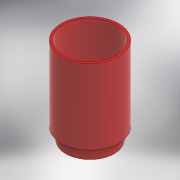
# Autodesk Inventor part: flour_duct
Saved by Autodesk Inventor 2020 (Build 240168000, 168)
## iProperties
Created: 2020-06-18
Part Number: flour_duct
Material: Generic
Document SubType Name: Modeling
Designer: pc-konvi
Density: 1 g/cm^3
Appearance: Red
Author: pc-konvi
Autodesk Inventor part; units mm, degrees
ref_plane "YZ Plane" through (0, 0, 0) normal (1, 0, 0) x (0, 1, 0)
ref_plane "XZ Plane" through (0, 0, 0) normal (0, 1, 0) x (-1, 0, 0)
ref_plane "XY Plane" through (0, 0, 0) normal (0, 0, 1) x (1, 0, 0)
sketch "Sketch1" plane through (0, 0, 0) normal (0, 0, 1) x (1, 0, 0)
  line L0 (0, 0) -> (25, 0) construction
  line L1 (25, 0) -> (25, 65) construction
  line L2 (25, 65) -> (0, 65) construction
  line L3 (0, 65) -> (0, 0) construction
  line L4 (25, 65) -> (23, 65)
  line L5 (23, 65) -> (23, 0)
  line L6 (23, 0) -> (25, 0)
  line L7 (25, 0) -> (25, 65)
  line L8 (0, 0) -> (21, 0) construction
  line L9 (21, 0) -> (21, -10) construction
  line L10 (21, -10) -> (0, -10) construction
  line L11 (0, -10) -> (0, 0) construction
  line L12 (21, 0) -> (19, 0)
  line L13 (19, 0) -> (19, -10)
  line L14 (19, -10) -> (21, -10)
  line L15 (21, -10) -> (21, 0)
  line L16 (19, 0) -> (25, 0)
  line L17 (25, 0) -> (25, 2)
  line L18 (25, 2) -> (19, 2)
  line L19 (19, 2) -> (19, 0)
  point P0 (23, 2)
  dimension "d0" = 25
  dimension "d1" = 65
  dimension "d2" = 2
  dimension "d3" = 21
  dimension "d4" = 10
  dimension "d5" = 2
  dimension "d6" = 2
  constraints: 40 end point, 10 parallel, 5 horizontal, 5 perpendicular, 3 point on line
  measures "d0" distance of L2.end L1.end
  measures "d1" distance of L1.end L0.end
  measures "d2" distance of L6.end L5.end
  measures "d3" distance of L9.end L10.end
  measures "d4" distance of L8.end L9.end
  measures "d5" distance of L14.end L13.end
  measures "d6" distance of L17.end L16.end
revolve "Revolution1" add sketch "Sketch1" angle 360 about axis through (0, 65, 0) along (0, -1, 0)
body "Solid1"
